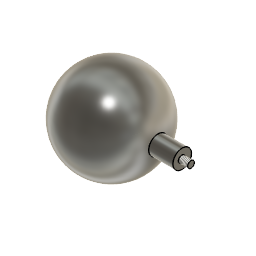
BRASPOURGLISSIERE (Autodesk Fusion 360 design; units mm, degrees)
Autodesk Fusion 360 part; units mm, degrees
sphere "SpherePrimitive1" add diameter 40 placed x (0, 1, 0) y (0, 0, 1) z (1, 0, 0) at (0, 0, 0)
cylinder "CylindrePrimitive1" add diameter 8 height 30 placed x (0, 0, -1) y (0, 1, 0) z (1, 0, 0) at (0, 0.2086, 0)
cylinder "CylindrePrimitive2" add diameter 3 height 4 placed x (0, 0, -1) y (0, 1, 0) z (1, 0, 0) at (30, 0, 0)
thread "Filetage1" "ISO Metric profile 3.0 M3x0.5 M3x0.5 6g" major diameter 2.927 minor diameter 2.3555 pitch 0.5 angle 60 resizes the face on face at (32.6667, -0.1494, -1.4925)
